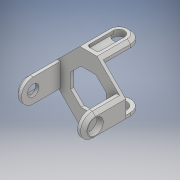
# Autodesk Inventor part: COXA2
Saved by Autodesk Inventor 2017 (Build 210142000, 142)
## iProperties
Created: 2017-09-24
Part Number: COXA2
Material: Generic
Document SubType Name: Modeling
Designer: Alexander Miller
Density: 1 g/cm^3
Appearance: Default
Author: Alexander Miller
Autodesk Inventor part; units mm, degrees
ref_plane "YZ Plane" through (0, 0, 0) normal (1, 0, 0) x (0, 1, 0)
ref_plane "XZ Plane" through (0, 0, 0) normal (0, 1, 0) x (-1, 0, 0)
ref_plane "XY Plane" through (0, 0, 0) normal (0, 0, 1) x (1, 0, 0)
sketch "Sketch1" plane through (0, 0, 0) normal (0, 1, 0) x (-1, 0, 0)
  line L0 (20, 7.5) -> (-20, 7.5) construction
  line L1 (-20, 7.5) -> (-20, -7.5)
  line L2 (-20, -7.5) -> (20, -7.5) construction
  line L3 (20, -7.5) -> (20, 7.5)
  line L4 (7.5, 20) -> (-7.5, 20)
  line L5 (-7.5, 20) -> (-7.5, -20) construction
  line L6 (-7.5, -20) -> (7.5, -20)
  line L7 (7.5, -20) -> (7.5, 20) construction
  line L8 (20, 7.5) -> (7.5, 20)
  line L9 (-7.5, 20) -> (-20, 7.5)
  line L10 (-20, -7.5) -> (-7.5, -20)
  line L11 (7.5, -20) -> (20, -7.5)
  point P0 (0, 0)
  point P1 (0, -7.5)
  point P2 (20, 0)
  point P3 (0, 20)
  point P4 (7.5, 0)
  dimension "d0" = 40
  dimension "d1" = 15
  constraints: 24 end point, 7 perpendicular, 4 midpoint, 4 parallel, 2 horizontal, 2 horizontal alignment, 2 vertical alignment
  measures "d0" distance of L1.end L2.end
  measures "d1" distance of L2.end L0.start
extrude "Extrusion1" add sketch "Sketch1" along normal blind 2
sketch "Sketch2" plane through (0, 0, 0) normal (0, -1, 0) x (1, 0, 0)
  line L0 (-20, 7.5) -> (-18, 7.5)
  line L1 (-18, 7.5) -> (-18, -7.5)
  line L2 (-18, -7.5) -> (-20, -7.5)
  line L3 (-20, -7.5) -> (-20, 7.5)
  line L4 (18, 7.5) -> (20, 7.5)
  line L5 (20, 7.5) -> (20, -7.5)
  line L6 (20, -7.5) -> (18, -7.5)
  line L7 (18, -7.5) -> (18, 7.5)
  line L8 (-20, 7.5) -> (-20, -7.5) projected
  line L9 (20, -7.5) -> (20, 7.5) projected
  point P0 (0, 0)
  point P1 (19, 7.5)
  point P2 (19, -7.5)
  point P3 (-19, -7.5)
  point P4 (-19, 7.5)
  dimension "d4" = 2
  constraints: 16 end point, 4 horizontal alignment, 4 midpoint, 4 parallel, 3 collinear, 2 horizontal, 2 perpendicular
  measures "d4" distance of L0.start L0.end
extrude "Extrusion2" add sketch "Sketch2" along normal blind 25
full round fillet "Fillet1" first side at (-19.3333, -8.3333, 7.5) centre faces at (-19.3333, -25, 2.5) second side at (-18.6667, -8.3333, -7.5)
full round fillet "Fillet2" first side at (19.3333, -8.3333, -7.5) centre faces at (19.3333, -25, 2.5) second side at (18.6667, -8.3333, 7.5)
sketch "Sketch3" plane through (0, 2, 0) normal (0, 1, 0) x (1, 0, 0)
  line L0 (-7.5, -20) -> (7.5, -20)
  line L1 (7.5, -20) -> (7.5, -18)
  line L2 (7.5, -18) -> (-7.5, -18)
  line L3 (-7.5, -18) -> (-7.5, -20)
  line L4 (-7.5, 18) -> (7.5, 18)
  line L5 (7.5, 18) -> (7.5, 20)
  line L6 (7.5, 20) -> (-7.5, 20)
  line L7 (-7.5, 20) -> (-7.5, 18)
  line L8 (-7.5, -20) -> (7.5, -20) projected
  line L9 (7.5, 20) -> (-7.5, 20) projected
  point P0 (0, 0)
  point P1 (-7.5, -19)
  point P2 (7.5, -19)
  point P3 (-7.5, 19)
  dimension "d7" = 2
  constraints: 16 end point, 4 parallel, 3 collinear, 3 midpoint, 3 vertical alignment, 2 horizontal, 2 perpendicular, 1 point on line
  measures "d7" distance of L2.end L0.start
extrude "Extrusion3" add sketch "Sketch3" along normal blind 25
full round fillet "Fillet3" first side at (7.5, 10.3333, 19.3333) centre faces at (2.5, 27, 19.3333) second side at (-7.5, 10.3333, 18.6667)
full round fillet "Fillet4" first side at (-7.5, 10.3333, -19.3333) centre faces at (2.5, 27, -18.6667) second side at (7.5, 10.3333, -18.6667)
sketch "Sketch4" plane through (20, 2, 7.5) normal (1, 0, 0) x (0, 0, -1)
  circle A0 centre (7.5, -19.5) radius 5
  arc A1 (0, -19.5) -> (15, -19.5) centre (7.5, -19.5) ccw projected
  point P0 (7.5, -2)
  dimension "d10" = 10
  constraints: 1 centre point, 1 concentric
  measures "d10" diameter of A0
extrude "Extrusion4" cut sketch "Sketch4" against normal up to surface (2 mm away)
sketch "Sketch5" plane through (7.5, 0, -20) normal (0, 0, -1) x (-1, 0, 0)
  circle A0 centre (7.5, 19.5) radius 5
  arc A1 (15, 19.5) -> (0, 19.5) centre (7.5, 19.5) ccw projected
  point P0 (7.5, 0)
  dimension "d13" = 10
  constraints: 1 centre point, 1 concentric
  measures "d13" diameter of A0
extrude "Extrusion5" cut sketch "Sketch5" against normal up to surface (2 mm away)
sketch "Sketch6" plane through (-20, 2, -7.5) normal (-1, 0, 0) x (0, 0, 1)
  circle A0 centre (7.5, -19.5) radius 3.625
  arc A1 (0, -19.5) -> (15, -19.5) centre (7.5, -19.5) ccw projected
  point P0 (7.5, -2)
  dimension "d16" = 7.25
  constraints: 1 centre point, 1 concentric
  measures "d16" diameter of A0
extrude "Extrusion6" cut sketch "Sketch6" against normal up to surface (2 mm away)
sketch "Sketch7" plane through (-7.5, 0, 20) normal (0, 0, 1) x (1, 0, 0)
  circle A0 centre (7.5, 19.5) radius 3.625
  arc A1 (15, 19.5) -> (0, 19.5) centre (7.5, 19.5) ccw projected
  point P0 (7.5, 0)
  dimension "d19" = 7.25
  constraints: 1 centre point, 1 concentric
  measures "d19" diameter of A0
extrude "Extrusion7" cut sketch "Sketch7" against normal up to surface (2 mm away)
sketch "Sketch13" plane through (-7.5, 0, 20) normal (0, 0, 1) x (1, 0, 0)
  line L0 (3.875, 19.5) -> (3.875, 2.5)
  line L1 (0, 2) -> (0, 19.5) projected
  line L2 (3.875, 2.5) -> (11.125, 2.5)
  circle A0 centre (7.5, 19.5) radius 3.625 projected
  arc A1 (15, 19.5) -> (0, 19.5) centre (7.5, 19.5) ccw projected
  line L3 (0, 2) -> (0, 19.5) projected
  line L4 (0, 0) -> (0, 2) projected
  line L5 (15, 0) -> (0, 0) projected
  line L6 (15, 0) -> (15, 2) projected
  line L7 (15, 2) -> (15, 19.5) projected
  circle A2 centre (7.5, 19.5) radius 3.625 projected
  line L8 (11.125, 2.5) -> (11.125, 19.5)
  arc A3 (11.125, 19.5) -> (3.875, 19.5) centre (7.5, 19.5) ccw
  point P0 (7.5, 0)
  point P1 (12, 0)
  point P2 (7.5, 2.5)
  dimension "d51" = 17
  constraints: 6 end point, 2 point on circle, 2 vertical, 1 centre point, 1 horizontal alignment, 1 midpoint, 1 parallel, 1 perpendicular, 1 vertical alignment, 2 other
  measures "d51" distance from line of L2 A1.centre
extrude "Extrusion13" add sketch "Sketch13" along normal blind 2
sketch "Sketch14" plane through (20, 2, 7.5) normal (1, 0, 0) x (0, 0, -1)
  circle A0 centre (7.5, -19.5) radius 5 projected
  arc A1 (0, -19.5) -> (15, -19.5) centre (7.5, -19.5) ccw projected
  line L0 (15, -2) -> (15, -19.5) projected
  line L1 (15, -2) -> (15, 0) projected
  line L2 (0, 0) -> (15, 0) projected
  line L3 (0, -2) -> (0, 0) projected
  line L4 (0, -2) -> (0, -19.5) projected
extrude "Extrusion14" add sketch "Sketch14" along normal blind 2
sketch "Sketch15" plane through (7.5, 0, -20) normal (0, 0, -1) x (-1, 0, 0)
  circle A0 centre (7.5, 19.5) radius 5 projected
  line L0 (0, 2) -> (0, 19.5) projected
  line L1 (0, 0) -> (0, 2) projected
  circle A1 centre (7.5, 19.5) radius 5 projected
  arc A2 (15, 19.5) -> (0, 19.5) centre (7.5, 19.5) ccw projected
  line L2 (0, 2) -> (0, 19.5) projected
  line L3 (0, 0) -> (0, 2) projected
  line L4 (15, 0) -> (0, 0) projected
  line L5 (15, 0) -> (15, 2) projected
  line L6 (15, 2) -> (15, 19.5) projected
extrude "Extrusion15" add sketch "Sketch15" along normal blind 2
sketch "Sketch16" plane through (-20, 2, -7.5) normal (-1, 0, 0) x (0, 0, 1)
  line L0 (11.125, -19.5) -> (11.125, -2.5)
  line L1 (11.125, -2.5) -> (3.875, -2.5)
  line L2 (3.875, -2.5) -> (3.875, -19.5)
  line L3 (0, -2) -> (0, -19.5) projected
  line L4 (0, 0) -> (15, 0) projected
  line L5 (15, -2) -> (15, -19.5) projected
  circle A0 centre (7.5, -19.5) radius 3.625 projected
  circle A1 centre (7.5, -19.5) radius 3.625 projected
  arc A2 (0, -19.5) -> (15, -19.5) centre (7.5, -19.5) ccw projected
  line L6 (15, -2) -> (15, -19.5) projected
  line L7 (15, -2) -> (15, 0) projected
  line L8 (0, 0) -> (15, 0) projected
  line L9 (0, -2) -> (0, 0) projected
  line L10 (0, -2) -> (0, -19.5) projected
  arc A3 (3.875, -19.5) -> (11.125, -19.5) centre (7.5, -19.5) ccw
  point P0 (7.5, -2)
  point P1 (7.5, -2.5)
  dimension "d60" = 17
  constraints: 6 end point, 2 perpendicular, 2 point on circle, 1 centre point, 1 horizontal alignment, 1 midpoint, 1 parallel, 1 vertical, 1 vertical alignment, 2 other
  measures "d60" distance of point (7.5, -2.5) point (7.5, -19.5)
extrude "Extrusion16" add sketch "Sketch16" along normal blind 2
chamfer "Chamfer5" distance 2 angle 45 12 edges at (-7.5, 9.75, -22) (0, 27, -22) (7.5, 9.75, -22) (-7.5, 9.75, 22) (0, 27, 22) (7.5, 9.75, 22) (-22, -7.75, 7.5) (-22, -25, 0) (-22, -7.75, -7.5) (22, -7.75, -7.5) (22, -25, 0) (22, -7.75, 7.5)
fillet "Fillet7" radius 1.75 4 edges at (3.625, 2.5, 21) (-3.625, 2.5, 21) (-21, -0.5, 3.625) (-21, -0.5, -3.625)
sketch "Sketch17" plane through (0, 2, 0) normal (0, 1, 0) x (1, 0, 0)
  line L0 (-11.4454, 4.7409) -> (-4.7409, 11.4454)
  line L1 (-4.7409, 11.4454) -> (4.7409, 11.4454)
  line L2 (4.7409, 11.4454) -> (11.4454, 4.7409)
  line L3 (11.4454, 4.7409) -> (11.4454, -4.7409)
  line L4 (11.4454, -4.7409) -> (4.7409, -11.4454)
  line L5 (4.7409, -11.4454) -> (-4.7409, -11.4454)
  line L6 (-4.7409, -11.4454) -> (-11.4454, -4.7409)
  line L7 (-11.4454, -4.7409) -> (-11.4454, 4.7409)
  line L8 (-7.5, -20) -> (-22, -5.5) projected
  point P0 (0, 0)
  point P1 (0, 0)
  dimension "d72" = 8
  constraints: 16 end point, 1 coincident, 17 other
  measures "d72" distance between parallel lines of L8 L6
extrude "Extrusion17" cut sketch "Sketch17" against normal through all
equation "\"d10\" = bearing_A"
equation "\"d13\" = bearing_A"
equation "\"d16\" = servo_hat_A"
equation "\"d19\" = servo_hat_A"
equation "\"bearing_A\" = 10"
equation "\"servo_hat_A\" = 7.25"
body "Solid1"
